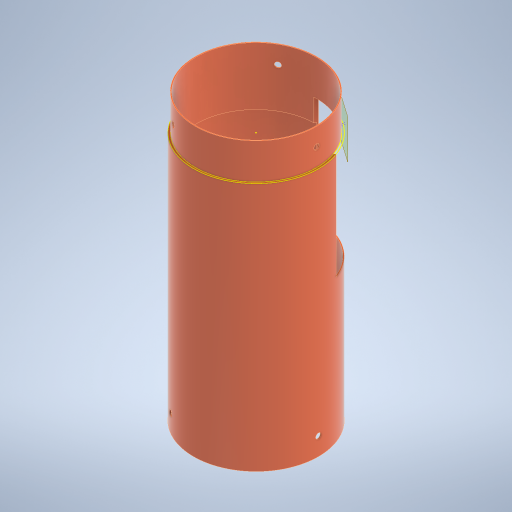
# Autodesk Inventor part: Lower skin
Saved by Autodesk Inventor 2024 (Build 280153000, 153)
## iProperties
Created: 2023-12-30
Part Number: Lower skin
Material: Plastic, Opaque White
Document SubType Name: Modeling
Designer: Jamie
Density: 0.952 g/cm^3
Appearance: Smooth - Light Orange
Author: Jamie
Autodesk Inventor part; units mm, degrees
ref_plane "XZ Plane" through (0, 0, 0) normal (0, 1, 0) x (-1, 0, 0)
ref_plane "XY Plane" through (0, 0, 0) normal (0, 0, 1) x (1, 0, 0)
sketch "Sketch1" plane through (0, 0, 0) normal (0, 1, 0) x (-1, 0, 0)
  circle A0 centre (0, 0) radius 35
  circle A1 centre (0, 0) radius 34.5
  dimension "d0" = 70
  dimension "d1" = 69
  constraints: 2 centre point, 2 coincident
  measures "d0" diameter of A0
  measures "d1" diameter of A1
extrude "Extrusion1" add sketch "Sketch1" along normal blind 140
ref_plane "Work Plane2" through (35, 0, 0) normal (1, 0, 0) x (0, 1, 0)
sketch "Sketch4" plane through (35, 0, 0) normal (1, 0, 0) x (0, 1, 0)
  line L0 (140, -35) -> (140, 35) projected
  point P0 (0, 0)
  point P1 (10, 0)
  dimension "d48" = 10
  measures "d48" distance of point (0, 0) point (10, 0)
hole "Hole2" at (35, 10, 0) direction (-1, 0, 0) diameter 3 depth 8 tip angle 118
sketch "Sketch5" plane through (0, 140, 0) normal (0, 1, 0) x (1, 0, 0)
  circle A0 centre (0, 0) radius 34
  circle A1 centre (0, 0) radius 33.5
  dimension "d44" = 68
  dimension "d45" = 67
  constraints: 2 centre point, 2 coincident
  measures "d44" diameter of A0
  measures "d45" diameter of A1
extrude "Extrusion3" add sketch "Sketch5" along normal blind 20
sketch "Sketch6" plane through (0, 140, 0) normal (0, -1, 0) x (1, 0, 0)
  circle A0 centre (0, 0) radius 33.5
  circle A1 centre (0, 0) radius 34.5 projected
  circle A2 centre (0, 0) radius 35
  constraints: 2 centre point, 2 coincident
extrude "Extrusion4" add sketch "Sketch6" along normal blind 12.5 contours A1
ref_plane "Work Plane4" through (34, 0, 0) normal (1, 0, 0) x (0, 1, 0)
sketch "Sketch8" plane through (34, 0, 0) normal (1, 0, 0) x (0, 1, 0)
  line L0 (160, -34) -> (160, 34) projected
  line L1 (150, 0) -> (50.9315, 0)
  line L2 (140, -35) -> (140, 35) projected
  line L3 (130, 15) -> (85, 15)
  line L4 (85, 15) -> (85, -15)
  line L5 (85, -15) -> (130, -15)
  line L6 (130, -15) -> (130, 15)
  point P0 (0, 0)
  point P1 (109.4746, 0)
  dimension "d61" = 10
  dimension "d74" = 15
  dimension "d75" = 10
  dimension "d76" = 15
  dimension "d77" = 55
  constraints: 10 end point, 3 horizontal, 2 parallel, 1 perpendicular
  measures "d61" distance from line of L0 L1.start
  measures "d74" distance from line of L1 L3.start
  measures "d75" distance from line of L2 L3.start
  measures "d76" distance from line of L1 L4.end
  measures "d77" distance from line of L2 L4.end
hole "Hole4" at (34, 150, 0) direction (-1, 0, 0) diameter 3 depth 8 tip angle 118
pattern_circular "Circular Pattern2" count 3 over 360 about axis through (0, 0, 0) along (0, 1, 0) of "Hole2", "Hole4"
sketch "Sketch9" plane through (0, 140, 0) normal (0, 1, 0) x (1, 0, 0)
  point P0 (0, 0)
sketch "Sketch10" plane through (0, 140, 0) normal (0, 1, 0) x (1, 0, 0)
  point P0 (0, 0)
sketch "Sketch13" plane through (0, 160, 0) normal (0, 1, 0) x (1, 0, 0)
  line L0 (0, 0) -> (41.3541, -71.6274) construction
  line L1 (47.0177, 0) -> (-69.3856, 0) construction
  circle A0 centre (0, 0) radius 35 projected
  point P0 (17.5, -30.3109)
  dimension "d87" = 60
  constraints: 4 end point, 1 horizontal, 1 point on line, 2 other
  measures "d87" angle of L1 L0
ref_plane "Work Plane6" through (17.5, 160, 30.3109) normal (0.5, 0, 0.8660254) x (0, 1, 0)
sketch "Sketch20" plane through (0, 140, 0) normal (0, 1, 0) x (1, 0, 0)
  circle A0 centre (0, 0) radius 34 projected
  circle A1 centre (0, 0) radius 35 projected
  point P0 (20.0284, 27.4748)
  point P1 (20.0284, 28.7031)
  constraints: 4 other
ref_plane "Work Plane9" through (20.0284, 140, -28.7031) normal (0.5722386, 0, -0.8200872) x (0, 1, 0)
sketch "Sketch21" plane through (20.0284, 140, -28.7031) normal (0.5722386, 0, -0.8200872) x (0, 1, 0)
  line L0 (0, -34) -> (0, 34) projected
  line L1 (0, 0) -> (-54.6676, 0) construction
  line L2 (0, 20) -> (-60, 20)
  line L3 (-60, 20) -> (-60, -20)
  line L4 (-60, -20) -> (0, -20)
  line L5 (0, -20) -> (0, 20)
  point P0 (-140, 0)
  point P1 (0, 20)
  dimension "d132" = 20
  dimension "d133" = 20
  dimension "d134" = 0
  dimension "d135" = 60
  constraints: 10 end point, 3 horizontal, 2 parallel, 1 midpoint, 1 perpendicular
  measures "d132" distance from line of L1 L3.end
  measures "d133" distance from line of L1 L2.start
  measures "d134" distance from line of L0 L2.start
  measures "d135" distance from line of L0 L3.end
extrude "Extrusion7" cut sketch "Sketch21" against normal blind 10
body "Solid1"
